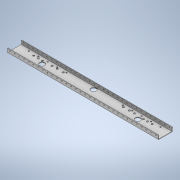
# Autodesk Inventor part: AM14U4_Plate
Saved by Autodesk Inventor 2020.3 (Build 243373000, 373)
## iProperties
Created: 2020-09-23
Part Number: AM14U4_Plate
Material: Generic
Document SubType Name: Modeling
Designer: super
Density: 1 g/cm^3
Appearance: Default
Author: super
Autodesk Inventor part; units mm, degrees
ref_plane "YZ Plane" through (0, 0, 0) normal (1, 0, 0) x (0, 1, 0)
ref_plane "XZ Plane" through (0, 0, 0) normal (0, 1, 0) x (-1, 0, 0)
ref_plane "XY Plane" through (0, 0, 0) normal (0, 0, 1) x (1, 0, 0)
sketch "Sketch1" plane through (0, 0, 0) normal (1, 0, 0) x (0, 1, 0)
  line L0 (0, 0) -> (-22.225, 0)
  line L1 (-22.225, 0) -> (-22.225, 77.724)
  line L2 (-22.225, 77.724) -> (0, 77.724)
  line L3 (0, 77.724) -> (0, 74.422)
  line L4 (0, 74.422) -> (-18.923, 74.422)
  line L5 (-18.923, 74.422) -> (-18.923, 3.302)
  line L6 (-18.923, 3.302) -> (0, 3.302)
  line L7 (0, 3.302) -> (0, 0)
  dimension "d0" = 22.225
  dimension "d1" = 77.724
  dimension "d2" = 3.302
  dimension "d3" = 18.923
  dimension "d4" = 71.12
  constraints: 16 end point, 7 perpendicular, 1 horizontal, 1 point on line
  measures "d0" distance of L0.start L0.end
  measures "d1" distance of L0.end L1.end
  measures "d2" distance of L2.end L3.end
  measures "d3" distance of L3.end L4.end
  measures "d4" distance of L4.end L5.end
extrude "Extrusion1" add sketch "Sketch1" against normal blind 812.8
fillet "Fillet1" radius 3.175 1 edges at (-406.4, -22.225, 0)
fillet "Fillet2" radius 3.175 1 edges at (-406.4, -22.225, 77.724)
sketch "Sketch2" plane through (0, 0, 0) normal (0, 0, -1) x (-1, 0, 0)
  circle A0 centre (12.7, -6.35) radius 2.667
  point P0 (0, 0)
  dimension "d11" = 5.334
  constraints: 1 centre point
  measures "d11" diameter of A0
extrude "Extrusion2" cut sketch "Sketch2" against normal blind 3.302
pattern_linear "Rectangular Pattern1" count 32 spacing 25.4 along (-1, 0, 0) of "Extrusion2"
sketch "Sketch3" plane through (-812.8, 0, 77.724) normal (0, 0, 1) x (1, 0, 0)
  line L0 (812.8, -18.923) -> (812.8, 0) projected
  circle A0 centre (800.1, -6.35) radius 2.667
  dimension "d19" = 5.334
  constraints: 1 centre point
  measures "d19" diameter of A0
extrude "Extrusion3" cut sketch "Sketch3" against normal blind 3.302
pattern_linear "Rectangular Pattern2" count 32 spacing 25.4 along (-1, 0, 0) of "Extrusion3"
sketch "Sketch4" plane through (-812.8, -22.225, 3.175) normal (0, -1, 0) x (1, 0, 0)
  line L0 (812.8, 71.374) -> (812.8, 0) projected
  line L1 (812.8, 74.549) -> (0, 74.549) projected
  circle A0 centre (406.4, 16.129) radius 14.2875
  line L2 (0, 71.374) -> (812.8, 71.374) projected
  line L3 (0, 0) -> (0, 71.374) projected
  point P0 (812.8, -3.175)
  dimension "d28" = 28.575
  dimension "d29" = 55.245
  dimension "d30" = 406.4
  constraints: 1 centre point
  measures "d28" diameter of A0
  measures "d29" distance from line of A0.centre L2
  measures "d30" distance from line of L3 A0.centre
extrude "Extrusion4" cut sketch "Sketch4" against normal blind 3.302
sketch "Sketch5" plane through (-812.8, -22.225, 3.175) normal (0, -1, 0) x (1, 0, 0)
  circle A0 centre (147.828, 35.687) radius 14.2875
  line L0 (0, 71.374) -> (812.8, 71.374) projected
  line L1 (0, 0) -> (0, 71.374) projected
  point P0 (812.8, -3.175)
  dimension "d33" = 28.575
  dimension "d34" = 35.687
  dimension "d35" = 147.828
  constraints: 1 centre point
  measures "d33" diameter of A0
  measures "d34" distance from line of L0 A0.centre
  measures "d35" distance from line of L1 A0.centre
extrude "Extrusion5" cut sketch "Sketch5" against normal blind 3.302
sketch "Sketch6" plane through (-812.8, -22.225, 3.175) normal (0, -1, 0) x (1, 0, 0)
  circle A0 centre (664.972, 35.687) radius 14.2875
  line L0 (0, 71.374) -> (812.8, 71.374) projected
  line L1 (812.8, 71.374) -> (812.8, 0) projected
  point P0 (812.8, -3.175)
  dimension "d38" = 28.575
  dimension "d39" = 35.687
  dimension "d40" = 147.828
  constraints: 1 centre point
  measures "d38" diameter of A0
  measures "d39" distance from line of A0.centre L0
  measures "d40" distance from line of L1 A0.centre
extrude "Extrusion6" cut sketch "Sketch6" against normal blind 3.302
sketch "Sketch7" plane through (-812.8, -22.225, 3.175) normal (0, -1, 0) x (1, 0, 0)
  circle A0 centre (50.8, 61.087) radius 3.3782
  line L0 (0, 71.374) -> (812.8, 71.374) projected
  line L1 (0, 0) -> (0, 71.374) projected
  point P0 (812.8, -3.175)
  dimension "d43" = 6.7564
  dimension "d44" = 10.287
  dimension "d45" = 50.8
  constraints: 1 centre point
  measures "d43" diameter of A0
  measures "d44" distance from line of L0 A0.centre
  measures "d45" distance from line of L1 A0.centre
extrude "Extrusion7" cut sketch "Sketch7" against normal blind 3.302
pattern_linear "Rectangular Pattern3" count 15 spacing 50.8 along (1, 0, 0) of "Extrusion7"
sketch "Sketch8" plane through (-812.8, -22.225, 3.175) normal (0, -1, 0) x (1, 0, 0)
  circle A0 centre (50.8, 10.287) radius 3.3782
  line L0 (0, 0) -> (0, 71.374) projected
  line L1 (812.8, 0) -> (0, 0) projected
  point P0 (812.8, -3.175)
  dimension "d51" = 6.7564
  dimension "d52" = 50.8
  dimension "d53" = 10.287
  constraints: 1 centre point
  measures "d51" diameter of A0
  measures "d52" distance from line of L0 A0.centre
  measures "d53" distance from line of L1 A0.centre
extrude "Extrusion8" cut sketch "Sketch8" against normal blind 3.302
pattern_linear "Rectangular Pattern4" count 5 spacing 50.8 along (1, 0, 0) of "Extrusion8"
sketch "Sketch9" plane through (-812.8, -22.225, 3.175) normal (0, -1, 0) x (1, 0, 0)
  circle A0 centre (762, 10.287) radius 3.3782
  line L0 (812.8, 71.374) -> (812.8, 0) projected
  line L1 (812.8, 0) -> (0, 0) projected
  point P0 (812.8, -3.175)
  dimension "d59" = 6.7564
  dimension "d60" = 50.8
  dimension "d61" = 10.287
  constraints: 1 centre point
  measures "d59" diameter of A0
  measures "d60" distance from line of L0 A0.centre
  measures "d61" distance from line of L1 A0.centre
extrude "Extrusion9" cut sketch "Sketch9" against normal blind 3.302
pattern_linear "Rectangular Pattern5" count 5 spacing 50.8 along (-1, 0, 0) of "Extrusion9"
sketch "Sketch10" plane through (-812.8, -22.225, 3.175) normal (0, -1, 0) x (1, 0, 0)
  circle A0 centre (583.5396, 61.087) radius 3.3782
  line L0 (0, 71.374) -> (812.8, 71.374) projected
  line L1 (812.8, 71.374) -> (812.8, 0) projected
  point P0 (812.8, -3.175)
  dimension "d67" = 6.7564
  dimension "d68" = 10.287
  dimension "d69" = 229.2604
  constraints: 1 centre point
  measures "d67" diameter of A0
  measures "d68" distance from line of L0 A0.centre
  measures "d69" distance from line of L1 A0.centre
extrude "Extrusion10" cut sketch "Sketch10" against normal blind 3.302
pattern_linear "Rectangular Pattern6" count 2 spacing 354.2792 along (-1, 0, 0) of "Extrusion10"
sketch "Sketch11" plane through (-812.8, -22.225, 3.175) normal (0, -1, 0) x (1, 0, 0)
  circle A0 centre (86.3346, 19.685) radius 4.826
  line L0 (812.8, 0) -> (0, 0) projected
  line L1 (0, 0) -> (0, 71.374) projected
  point P0 (812.8, -3.175)
  dimension "d75" = 9.652
  dimension "d76" = 19.685
  dimension "d77" = 86.3346
  constraints: 1 centre point
  measures "d75" diameter of A0
  measures "d76" distance from line of L0 A0.centre
  measures "d77" distance from line of L1 A0.centre
extrude "Extrusion11" cut sketch "Sketch11" against normal blind 3.302
pattern_linear "Rectangular Pattern7" count 2 spacing 25.019 along (1, 0, 0) of "Extrusion11"
pattern_linear "Rectangular Pattern8" count 2 spacing 47.5234 along (1, 0, 0) of "Extrusion11"
sketch "Sketch12" plane through (-812.8, -22.225, 3.175) normal (0, -1, 0) x (1, 0, 0)
  circle A0 centre (183.8452, 17.907) radius 4.826
  line L0 (812.8, 0) -> (0, 0) projected
  line L1 (0, 0) -> (0, 71.374) projected
  point P0 (812.8, -3.175)
  dimension "d86" = 9.652
  dimension "d87" = 17.907
  dimension "d88" = 183.8452
  constraints: 1 centre point
  measures "d86" diameter of A0
  measures "d87" distance from line of L0 A0.centre
  measures "d88" distance from line of L1 A0.centre
extrude "Extrusion12" cut sketch "Sketch12" against normal blind 3.302
pattern_linear "Rectangular Pattern9" count 2 spacing 27.5082 along (1, 0, 0) of "Extrusion12"
pattern_linear "Rectangular Pattern10" count 2 spacing 60.0202 along (1, 0, 0) of "Extrusion12"
sketch "Sketch13" plane through (-812.8, -22.225, 3.175) normal (0, -1, 0) x (1, 0, 0)
  circle A0 centre (726.4654, 19.685) radius 4.826
  line L0 (812.8, 71.374) -> (812.8, 0) projected
  line L1 (812.8, 0) -> (0, 0) projected
  point P0 (812.8, -3.175)
  dimension "d97" = 9.652
  dimension "d98" = 86.3346
  dimension "d99" = 19.685
  constraints: 1 centre point
  measures "d97" diameter of A0
  measures "d98" distance from line of L0 A0.centre
  measures "d99" distance from line of L1 A0.centre
extrude "Extrusion13" cut sketch "Sketch13" against normal blind 3.302
pattern_linear "Rectangular Pattern11" count 2 spacing 25.019 along (-1, 0, 0) of "Extrusion13"
pattern_linear "Rectangular Pattern12" count 2 spacing 47.5234 along (-1, 0, 0) of "Extrusion13"
sketch "Sketch14" plane through (-812.8, -22.225, 3.175) normal (0, -1, 0) x (1, 0, 0)
  circle A0 centre (628.9548, 17.907) radius 4.826
  line L0 (812.8, 71.374) -> (812.8, 0) projected
  line L1 (812.8, 0) -> (0, 0) projected
  point P0 (812.8, -3.175)
  dimension "d108" = 9.652
  dimension "d109" = 183.8452
  dimension "d110" = 17.907
  constraints: 1 centre point
  measures "d108" diameter of A0
  measures "d109" distance from line of L0 A0.centre
  measures "d110" distance from line of L1 A0.centre
extrude "Extrusion14" cut sketch "Sketch14" against normal blind 3.302
pattern_linear "Rectangular Pattern13" count 2 spacing 27.5082 along (-1, 0, 0) of "Extrusion14"
pattern_linear "Rectangular Pattern14" count 2 spacing 60.0202 along (-1, 0, 0) of "Extrusion14"
body "Solid1"
